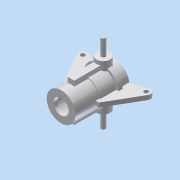
# Autodesk Inventor part: Axle Body - Front - Custom
Saved by Autodesk Inventor 2011 SP1 (Build 150282100, 282)
## iProperties
Created: 2011-09-22
Part Number: Axle Body - Front - Custom
Document SubType Name: Modeling
Designer: dgitz
Density: 1 g/cm^3
Author: dgitz
Autodesk Inventor part; units mm, degrees
sketch "Sketch2" plane through (0, 0, 0) normal (0, 0, 1) x (1, 0, 0)
  circle A0 centre (0, 0) radius 8.382
  dimension "d0" = 16.764
  constraints: 1 centre point, 1 coincident
  measures "d0" diameter of A0
extrude "Extrusion1" add sketch "Sketch2" along normal blind 13.97
sketch "Sketch3" plane through (0, 0, 0) normal (0, 0, -1) x (-1, 0, 0)
  circle A0 centre (0, 0) radius 8.382 projected
  circle A1 centre (0, 0) radius 8.89
  dimension "d3" = 17.78
  constraints: 1 centre point, 1 coincident
  measures "d3" diameter of A1
extrude "Extrusion2" add sketch "Sketch3" along normal blind 17.018 contours A0 | A1
ref_plane "Work Plane1" through (0, 0, -9.398) normal (0, 0, 1) x (1, 0, 0)
sketch "Sketch4" plane through (0, 0, -9.398) normal (0, 0, 1) x (1, 0, 0)
  circle A0 centre (0, 0) radius 8.89
  circle A1 centre (0, 0) radius 10.287
  circle A2 centre (0, 0) radius 8.89 projected
  dimension "d7" = 20.574
  constraints: 2 centre point, 2 coincident, 1 concentric
  measures "d7" diameter of A1
extrude "Extrusion3" add sketch "Sketch4" against normal blind 2.54
ref_plane "Work Plane6" through (0, 13.462, 0) normal (0, 1, 0) x (-1, 0, 0)
ref_plane "Work Plane5" through (0, 8.89, 0) normal (0, 1, 0) x (-1, 0, 0)
sketch "Sketch6" plane through (0, 13.462, 0) normal (0, 1, 0) x (-1, 0, 0)
  circle A0 centre (0, -10.668) radius 3.937
  line L0 (-9.4933, -9.398) -> (9.4933, -9.398) projected
  line L1 (9.4933, -11.938) -> (-9.4933, -11.938) projected
  line L2 (0, -24.5018) -> (0, -30.8914) construction
  point P0 (0, 0)
  dimension "d16" = 7.874
  dimension "d17" = 1.27
  constraints: 2 end point, 1 centre point, 1 perpendicular, 1 point on line
  measures "d16" diameter of A0
  measures "d17" distance from line of A0.centre L0
extrude "Extrusion4" add sketch "Sketch6" against normal up to surface
ref_plane "Work Plane7" through (0, 0, 8.128) normal (0, 0, 1) x (1, 0, 0)
sketch "Sketch7" plane through (0, 0, 8.128) normal (0, 0, 1) x (1, 0, 0)
  circle A0 centre (0, 0) radius 8.382 projected
  line L0 (-1.905, 8.1627) -> (-1.905, 11.2107)
  line L1 (-1.905, 11.2107) -> (1.905, 11.2107)
  line L2 (1.905, 11.2107) -> (1.905, 8.1627)
  arc A1 (1.905, 8.1627) -> (-1.905, 8.1627) centre (0, 0) ccw
  dimension "d25" = 16.764
  dimension "d26" = 3.81
  dimension "d27" = 3.048
  dimension "d28" = 1.905
  constraints: 6 end point, 2 point on circle, 1 centre point, 1 concentric, 1 horizontal, 1 parallel, 1 perpendicular
  measures "d25" diameter of A1
  measures "d26" distance between parallel lines of L2 L0
  measures "d27" distance from line of L0.start L1
  measures "d28" distance from line of A1.centre L0
extrude "Extrusion5" add sketch "Sketch7" against normal up to surface contours A0 L0 L1 L2
pattern_circular "Circular Pattern1" count 2 over 360 about axis through (0, 0, 0) along (0, 0, 1) of "Extrusion4", "Extrusion5"
sketch "Sketch8" plane through (0, 13.462, -10.668) normal (0, 1, 0) x (1, 0, 0)
  circle A0 centre (0, 0) radius 3.937 projected
  circle A1 centre (0, 0) radius 1.27
  point P0 (0, -10.668)
  dimension "d34" = 2.54
  constraints: 1 centre point, 1 coincident
  measures "d34" diameter of A1
extrude "Extrusion6" add sketch "Sketch8" along normal blind 9.525 contours A1
pattern_circular "Circular Pattern2" count 2 over 360 about axis through (0, 0, 0) along (0, 0, 1) of "Extrusion6"
sketch "Sketch9" plane through (0, 0, -17.018) normal (0, 0, -1) x (-1, 0, 0)
  circle A0 centre (0, 0) radius 8.89 projected
  circle A1 centre (0, 0) radius 6.985
  dimension "d40" = 13.97
  constraints: 1 centre point, 1 coincident
  measures "d40" diameter of A1
extrude "Extrusion7" cut sketch "Sketch9" against normal blind 28.448 contours A1
sketch "Sketch10" plane through (0, 0, 13.97) normal (0, 0, 1) x (1, 0, 0)
  circle A0 centre (0, 0) radius 8.382 projected
  circle A1 centre (0, 0) radius 4.445
  dimension "d43" = 8.89
  constraints: 1 centre point, 1 coincident
  measures "d43" diameter of A1
extrude "Extrusion8" cut sketch "Sketch10" against normal up to surface (2.54 mm away) contours A1
sketch "Sketch12" plane through (0, 0, 0) normal (0, 1, 0) x (-1, 0, 0)
  line L0 (-10.287, -17.018) -> (-10.287, 2.032)
  circle A0 centre (-18.4993, -17.2721) radius 1.27
  arc A1 (-20.699, -16.0021) -> (-17.6397, -19.6623) centre (-18.4993, -17.2721) ccw
  line L1 (-10.287, 2.032) -> (-20.699, -16.0021)
  line L2 (-10.287, -17.018) -> (-17.6397, -19.6623)
  line L3 (8.89, -17.018) -> (-8.89, -17.018) projected
  line L4 (-10.287, -9.398) -> (-10.287, -11.938) projected
  line L5 (0, -20.2977) -> (0, -33.1857) construction
  line L6 (10.287, -17.018) -> (10.287, 2.032)
  circle A2 centre (18.4993, -17.2721) radius 1.27
  arc A3 (17.6397, -19.6623) -> (20.699, -16.0021) centre (18.4993, -17.2721) ccw
  line L7 (10.287, 2.032) -> (20.699, -16.0021)
  line L8 (10.287, -17.018) -> (17.6397, -19.6623)
  line L9 (10.287, -9.398) -> (10.287, -11.938)
  point P0 (0, 0)
  dimension "d46" = 2.54
  dimension "d47" = 5.08
  dimension "d48" = 30
  dimension "d49" = 19.05
  constraints: 16 end point, 8 symmetric about line, 4 centre point, 4 point on circle, 2 coincident, 2 tangent, 1 collinear, 1 parallel, 1 point on line, 1 vertical, 2 other
  measures "d46" diameter of A0
  measures "d47" diameter of A1
  measures "d48" angle of L0 L1
  measures "d49" distance of L0.start L0.end
extrude "Extrusion9" add sketch "Sketch12" along normal mid plane 2.54
sketch "Sketch13" plane through (10.287, -1.27, -17.018) normal (-1, 0, 0) x (0, 0, 1)
  line L0 (0, 2.54) -> (19.05, 2.54)
  line L1 (19.05, 2.54) -> (19.05, 0)
  line L2 (19.05, 0) -> (0, 0)
  line L3 (0, 0) -> (0, 2.54)
  point P0 (17.018, 1.27)
  constraints: 8 end point, 2 parallel, 1 horizontal, 1 perpendicular
extrude "Extrusion10" add sketch "Sketch13" along normal up to surface
mirror "Mirror1" about plane through (0, 0, 0) normal (1, 0, 0) of "Extrusion10"
body "Solid1"
